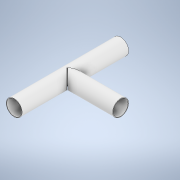
# Autodesk Inventor part: вставка в трубу
Saved by Autodesk Inventor 2020.1 (Build 241239000, 239)
## iProperties
Created: 2021-07-14
Part Number: вставка в трубу
Material: Полистирол, высокопрочный
Document SubType Name: Modeling
Designer: Ni3na
Density: 1.022 g/cm^3
Appearance: Гладкий — белый
Author: Ni3na
Autodesk Inventor part; units mm, degrees
ref_plane "YZ Plane" through (0, 0, 0) normal (1, 0, 0) x (0, 1, 0)
ref_plane "XZ Plane" through (0, 0, 0) normal (0, 1, 0) x (-1, 0, 0)
ref_plane "XY Plane" through (0, 0, 0) normal (0, 0, 1) x (1, 0, 0)
sketch "Эскиз1" plane through (0, 0, 0) normal (0, 0, 1) x (1, 0, 0)
  line L0 (0, 0) -> (150, 0)
  line L1 (150, 0) -> (150, -150)
  line L2 (150, -150) -> (0, -150)
  line L3 (0, -150) -> (0, 0)
  dimension "d0" = 150
  dimension "d1" = 150
  constraints: 8 end point, 2 parallel, 1 horizontal, 1 perpendicular
  measures "d0" distance of L0.start L0.end
  measures "d1" distance of L2.end L0.start
extrude "Выдавливание1" add sketch "Эскиз1" along normal blind 1000
sketch "Эскиз2" plane through (150, -150, 0) normal (1, 0, 0) x (0, 0, -1)
  line L0 (0, 0) -> (-1000, 0) projected
  line L1 (0, 150) -> (-1000, 150) projected
  line L2 (-575, 0) -> (-425, 0)
  line L3 (-425, 0) -> (-425, 150)
  line L4 (-425, 150) -> (-575, 150)
  line L5 (-575, 150) -> (-575, 0)
  point P0 (-500, 0)
  point P1 (-500, 0)
  point P2 (-425, 0)
  dimension "d4" = 150
  dimension "d5" = 0
  constraints: 8 end point, 2 midpoint, 2 parallel, 2 point on line, 1 horizontal, 1 perpendicular
  measures "d4" distance of L4.end L3.end
  measures "d5" distance of point (-500, 0) point (-500, 0)
extrude "Выдавливание2" add sketch "Эскиз2" along normal blind 425
sketch "Эскиз3" plane through (0, 0, 0) normal (0, 1, 0) x (1, 0, 0)
  line L0 (150, -425) -> (575, -425) projected
  line L1 (150, -575) -> (575, -575) projected
  line L2 (150, -425) -> (150, -575)
  line L3 (150, -500) -> (0, -500)
  line L4 (0, 0) -> (0, -1000) projected
  line L5 (75, -500) -> (150, -575)
  line L6 (80, -500) -> (155, -575)
  line L7 (70, -500) -> (150, -580)
  line L8 (150, -575) -> (150, -1000) projected
  circle A0 centre (77.5, -502.5) radius 3.5355
  point P0 (150, -570)
  point P1 (75, -505)
  dimension "d8" = 5
  dimension "d9" = 5
  constraints: 10 end point, 5 point on line, 3 midpoint, 2 parallel, 1 vertical, 3 other
  measures "d8" distance of L7.start L5.start
  measures "d9" distance of L5.start L6.start
extrude "Выдавливание3" cut sketch "Эскиз3" against normal blind 200 contours L2 L6 L1 | L5 A0 L6 L2 | L8 L7 A0 L5 | A0 L5 | L5 L3 A0 | L3 A0
fillet "Сопряжение1" radius 75 10 edges at (365, 0, 575) (362.5, 0, 425) (365, -150, 575) (362.5, -150, 425) (150, -150, 212.5) (150, 0, 212.5) (150, 0, 790) (150, -150, 790) (0, -150, 500) (0, 0, 500)
sketch "Эскиз4" plane through (75, -75, 1000) normal (0, 0, 1) x (1, 0, 0)
  line L0 (0, 75) -> (0, -75) projected
  circle A0 centre (0, 0) radius 70
  point P0 (-75, 75)
  dimension "d13" = 140
  constraints: 1 centre point, 1 midpoint
  measures "d13" diameter of A0
extrude "Выдавливание4" cut sketch "Эскиз4" against normal blind 1010
sketch "Эскиз5" plane through (575, -75, 500) normal (1, 0, 0) x (0, 0, -1)
  circle A0 centre (0, 0) radius 70
  point P0 (500, 75)
  dimension "d16" = 140
  constraints: 1 centre point
  measures "d16" diameter of A0
extrude "Выдавливание5" cut sketch "Эскиз5" against normal blind 500
